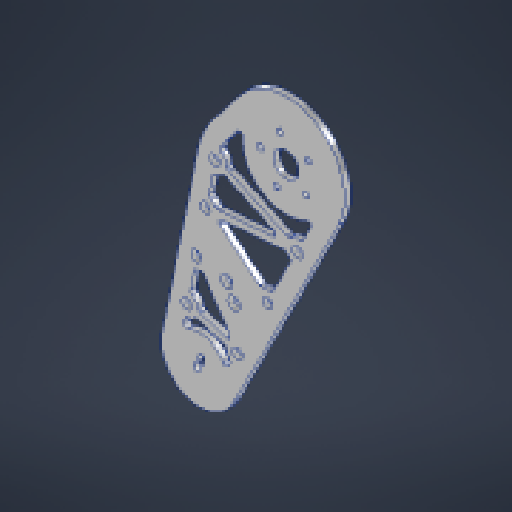
# Autodesk Inventor part: tank_inside_panel
Saved by Autodesk Inventor 2023 (Build 270158000, 158)
## iProperties
Created: 2023-02-28
Part Number: tank_inside_panel
Material: Aluminum 6061
Document SubType Name: Modeling
Designer: ralph
Density: 2.7 g/cm^3
Appearance: Aluminum - Flat
Author: ralph
Autodesk Inventor part; units mm, degrees
(part 1 of 3)
ref_plane "YZ Plane" through (0, 0, 0) normal (1, 0, 0) x (0, 1, 0)
ref_plane "XZ Plane" through (0, 0, 0) normal (0, 1, 0) x (-1, 0, 0)
ref_plane "XY Plane" through (0, 0, 0) normal (0, 0, 1) x (1, 0, 0)
sketch "Sketch1" plane through (0, 0, 0) normal (0, 0, 1) x (1, 0, 0)
  circle A0 centre (-51.8103, -146.0138) radius 3.175 projected
  circle A1 centre (-68.3289, -153.0646) radius 3.175 projected
  line L0 (-87.8938, -227.3235) -> (-92.6277, -239.1082) projected
  arc A2 (-98.5201, -236.7413) -> (-92.6277, -239.1082) centre (-95.5739, -237.9247) ccw projected
  line L1 (-98.5201, -236.7413) -> (-93.7862, -224.9565) projected
  arc A3 (-87.8938, -227.3235) -> (-93.7862, -224.9565) centre (-90.84, -226.14) ccw projected
  circle A4 centre (0, 0) radius 13.4937 projected
  line L2 (-56.4256, -250.7609) -> (56.5867, -28.8131) projected
  arc A5 (56.5867, -28.8131) -> (-50.0844, 39.0359) centre (0, 0) ccw projected
  line L3 (-50.0844, 39.0359) -> (-79.8174, 0.8875) projected
  arc A6 (-79.8174, 0.8875) -> (-94.3869, -30.7665) centre (-19.7161, -45.9556) ccw projected
  line L4 (-94.3869, -30.7665) -> (-133.6537, -223.8049) projected
  arc A7 (-133.6537, -223.8049) -> (-56.4256, -250.7609) centre (-93.207, -232.0324) ccw projected
  circle A8 centre (-6.7845, 27.1038) radius 3.175 projected
  circle A9 centre (-27.8737, 1.9231) radius 3.175 projected
  circle A10 centre (23.6807, 14.828) radius 3.175 projected
  circle A11 centre (-10.4424, -25.9152) radius 3.175 projected
  circle A12 centre (21.42, -17.9396) radius 3.175 projected
  circle A13 centre (12.3657, -76.0454) radius 2.413 projected
  circle A14 centre (-19.9049, -139.4226) radius 2.413 projected
  circle A15 centre (-52.1756, -202.7997) radius 2.413 projected
  line L5 (-60.0739, -215.9422) -> (-61.8764, -219.4822) projected
  arc A16 (-67.5559, -219.4407) -> (-61.8764, -219.4822) centre (-64.7057, -218.0416) ccw projected
  arc A17 (-109.9229, -202.7119) -> (-105.4512, -206.2136) centre (-106.8116, -203.3448) ccw projected
  line L6 (-109.9229, -202.7119) -> (-109.1463, -198.894) projected
  arc A18 (-106.2582, -196.3597) -> (-109.1463, -198.894) centre (-106.035, -199.5269) ccw projected
  arc A19 (-106.2582, -196.3597) -> (-98.2131, -192.7137) centre (-107.1508, -183.6911) ccw projected
  line L7 (4.4674, -89.1879) -> (-13.9226, -125.3045) projected
  arc A20 (-64.7826, -204.3336) -> (-60.7577, -212.1612) centre (-52.1756, -202.7997) ccw projected
  arc A21 (-60.0739, -215.9422) -> (-60.7577, -212.1612) centre (-62.9032, -214.5015) ccw projected
  arc A22 (-92.9225, -119.1363) -> (-91.2539, -122.5975) centre (-89.8112, -119.7692) ccw projected
  line L8 (-92.9225, -119.1363) -> (-88.8942, -99.3329) projected
  arc A23 (-86.006, -96.7986) -> (-88.8942, -99.3329) centre (-85.7829, -99.9658) ccw projected
  arc A24 (-86.006, -96.7986) -> (-81.66, -95.6992) centre (-86.8987, -84.1301) ccw projected
  arc A25 (-82.7964, -69.3558) -> (-81.1278, -72.8169) centre (-79.6851, -69.9886) ccw projected
  line L9 (-82.7964, -69.3558) -> (-78.7681, -49.5524) projected
  arc A26 (-75.88, -47.0181) -> (-78.7681, -49.5524) centre (-75.6568, -50.1853) ccw projected
  arc A27 (-64.0747, -34.1201) -> (-69.5394, -23.9106) centre (-76.7726, -34.3495) ccw projected
  arc A28 (-70.5555, -19.8506) -> (-69.5394, -23.9106) centre (-67.7311, -21.3009) ccw projected
  arc A29 (-64.7921, -10.8233) -> (-70.5555, -19.8506) centre (-19.7161, -45.9556) ccw projected
  line L10 (-64.7921, -10.8233) -> (-52.5862, 4.8373) projected
  arc A30 (-46.9122, 2.7029) -> (-52.5862, 4.8373) centre (-50.0819, 2.8855) ccw projected
  arc A31 (-46.9122, 2.7029) -> (-23.4162, -40.7399) centre (0, 0) ccw projected
  arc A32 (26.6737, -45.5765) -> (22.3352, -41.3425) centre (23.8443, -44.1359) ccw projected
  line L11 (26.6737, -45.5765) -> (18.3481, -61.9274) projected
  arc A33 (14.8881, -63.5984) -> (18.3481, -61.9274) centre (15.5187, -60.4867) ccw projected
  arc A34 (1.4524, -82.5408) -> (3.7836, -85.4069) centre (12.3657, -76.0454) ccw projected
  arc A35 (4.4674, -89.1879) -> (3.7836, -85.4069) centre (1.6381, -87.7473) ccw projected
  arc A36 (-17.3825, -126.9756) -> (-13.9226, -125.3045) centre (-16.7519, -123.8638) ccw projected
  arc A37 (-17.3825, -126.9756) -> (-25.1437, -127.8534) centre (-19.9049, -139.4226) ccw projected
  arc A38 (-63.388, -164.764) -> (-63.3432, -164.745) centre (-68.3289, -153.0646) ccw projected
  line L12 (-63.3432, -164.745) -> (-46.8246, -157.6942) projected
  arc A39 (-46.8246, -157.6942) -> (-39.1239, -145.4255) centre (-51.8103, -146.0138) ccw projected
  arc A40 (-35.726, -142.1115) -> (-39.1239, -145.4255) centre (-35.9523, -145.2784) ccw projected
  line L13 (-35.726, -142.1115) -> (-34.396, -142.2066) projected
  arc A41 (-31.6788, -144.1833) -> (-34.396, -142.2066) centre (-34.6223, -145.3735) ccw projected
  arc A42 (-31.6788, -144.1833) -> (-28.487, -148.784) centre (-19.9049, -139.4226) ccw projected
  arc A43 (-27.8032, -152.5651) -> (-28.487, -148.784) centre (-30.6326, -151.1244) ccw projected
  line L14 (-27.8032, -152.5651) -> (-46.1932, -188.6816) projected
  arc A44 (-49.6531, -190.3527) -> (-46.1932, -188.6816) centre (-49.0225, -187.241) ccw projected
  arc A45 (-49.6531, -190.3527) -> (-50.0187, -190.2842) centre (-52.1756, -202.7997) ccw projected
  arc A46 (-52.1403, -188.8876) -> (-50.0187, -190.2842) centre (-49.4795, -187.1553) ccw projected
  line L15 (-52.1403, -188.8876) -> (-64.8136, -169.4212) projected
  arc A47 (-63.388, -164.764) -> (-64.8136, -169.4212) centre (-62.1528, -167.6889) ccw projected
  arc A48 (-49.8906, -133.4597) -> (-51.925, -133.3143) centre (-51.8103, -146.0138) ccw projected
  line L16 (-51.925, -133.3143) -> (-82.5337, -131.1266) projected
  arc A49 (-85.2508, -129.1499) -> (-82.5337, -131.1266) centre (-82.3074, -127.9597) ccw projected
  arc A50 (-85.2508, -129.1499) -> (-91.2539, -122.5975) centre (-97.0248, -133.9106) ccw projected
  line L17 (-78.3293, -96.1428) -> (-39.1869, -128.4485) projected
  arc A51 (-41.4343, -134.0641) -> (-39.1869, -128.4485) centre (-41.2079, -130.8972) ccw projected
  line L18 (-41.4343, -134.0641) -> (-49.8906, -133.4597) projected
  line L19 (-94.9362, -191.9703) -> (-86.0453, -195.0607) projected
  arc A52 (-64.7826, -204.3336) -> (-66.8919, -201.7181) centre (-67.9343, -204.7171) ccw projected
  arc A53 (-94.9362, -191.9703) -> (-98.2131, -192.7137) centre (-95.9786, -194.9693) ccw projected
  line L20 (-65.4741, -43.8408) -> (-13.0902, -68.3442) projected
  arc A54 (-14.1778, -74.3847) -> (-13.0902, -68.3442) centre (-14.4355, -71.2201) ccw projected
  line L21 (-14.1778, -74.3847) -> (-72.9993, -79.1754) projected
  arc A55 (-75.9854, -77.6347) -> (-72.9993, -79.1754) centre (-73.2571, -76.0109) ccw projected
  arc A56 (-75.9854, -77.6347) -> (-81.1278, -72.8169) centre (-86.8987, -84.1301) ccw projected
  arc A57 (-65.4741, -43.8408) -> (-68.81, -44.2433) centre (-66.8194, -46.7167) ccw projected
  line L22 (-28.4744, -127.4098) -> (-71.2033, -92.144) projected
  arc A58 (-69.4401, -86.5307) -> (-71.2033, -92.144) centre (-69.1823, -89.6953) ccw projected
  line L23 (-69.4401, -86.5307) -> (-1.5337, -81.0001) projected
  arc A59 (1.4524, -82.5408) -> (-1.5337, -81.0001) centre (-1.2759, -84.1646) ccw projected
  arc A60 (-28.4744, -127.4098) -> (-25.1437, -127.8534) centre (-26.4534, -124.9611) ccw projected
  arc A61 (14.8881, -63.5984) -> (4.4031, -66.1517) centre (12.3657, -76.0454) ccw projected
  arc A62 (1.0672, -66.5541) -> (4.4031, -66.1517) centre (2.4124, -63.6782) ccw projected
  line L24 (1.0672, -66.5541) -> (-16.1602, -58.4958) projected
  arc A63 (-64.0747, -34.1201) -> (-62.2455, -36.9386) centre (-60.9002, -34.0627) ccw projected
  arc A64 (-61.0933, -193.7573) -> (-61.1133, -193.7771) centre (-52.1756, -202.7997) ccw projected
  arc A65 (-64.3902, -194.5205) -> (-61.1133, -193.7771) centre (-63.3478, -191.5215) ccw projected
  line L25 (-64.3902, -194.5205) -> (-92.4345, -184.7727) projected
  arc A66 (-94.5438, -182.1572) -> (-92.4345, -184.7727) centre (-91.3921, -181.7737) ccw projected
  arc A67 (-94.5438, -182.1572) -> (-101.38, -172.378) centre (-107.1508, -183.6911) ccw projected
  arc A68 (-103.0485, -168.9169) -> (-101.38, -172.378) centre (-99.9372, -169.5497) ccw projected
  line L26 (-103.0485, -168.9169) -> (-99.0202, -149.1135) projected
  arc A69 (-96.1321, -146.5792) -> (-99.0202, -149.1135) centre (-95.909, -149.7463) ccw projected
  arc A70 (-96.1321, -146.5792) -> (-92.3643, -145.7246) centre (-97.0248, -133.9106) ccw projected
  arc A71 (-88.5384, -146.9458) -> (-92.3643, -145.7246) centre (-91.1992, -148.6781) ccw projected
  line L27 (-88.5384, -146.9458) -> (-60.6619, -189.7645) projected
  arc A72 (-61.0933, -193.7573) -> (-60.6619, -189.7645) centre (-63.3227, -191.4968) ccw projected
  arc A73 (-88.6501, -203.823) -> (-105.4512, -206.2136) centre (-93.207, -232.0324) ccw projected
  line L28 (-22.0522, -44.6761) -> (-24.5423, -50.875) projected
  line L29 (-28.8338, -52.5675) -> (-62.2455, -36.9386) projected
  line L30 (-84.1415, -199.2432) -> (-85.1976, -201.8722) projected
  line L31 (-17.7611, -54.4364) -> (-14.9814, -47.5164) projected
  line L32 (-72.8348, -199.6524) -> (-66.8919, -201.7181) projected
  arc A74 (-67.5559, -219.4407) -> (-76.9832, -208.5096) centre (-93.207, -232.0324) ccw projected
  arc A75 (-75.88, -47.0181) -> (-68.81, -44.2433) centre (-76.7726, -34.3495) ccw projected
  line L33 (-78.1267, -204.7125) -> (-76.8234, -201.468) projected
  arc A76 (-11.2735, -45.6176) -> (22.3352, -41.3425) centre (0, 0) ccw projected
  arc A77 (-84.1415, -199.2432) -> (-86.0453, -195.0607) centre (-87.0877, -198.0597) ccw projected
  arc A78 (-88.6501, -203.823) -> (-85.1976, -201.8722) centre (-88.1438, -200.6887) ccw projected
  arc A79 (-22.0522, -44.6761) -> (-23.4162, -40.7399) centre (-24.9984, -43.4926) ccw projected
  arc A80 (-28.8338, -52.5675) -> (-24.5423, -50.875) centre (-27.4885, -49.6916) ccw projected
  arc A81 (-78.3293, -96.1428) -> (-81.66, -95.6992) centre (-80.3503, -98.5915) ccw projected
  arc A82 (-72.8348, -199.6524) -> (-76.8234, -201.468) centre (-73.8772, -202.6514) ccw projected
  arc A83 (-78.1267, -204.7125) -> (-76.9832, -208.5096) centre (-75.1805, -205.896) ccw projected
  arc A84 (-11.2735, -45.6176) -> (-14.9814, -47.5164) centre (-12.0352, -48.6999) ccw projected
  arc A85 (-17.7611, -54.4364) -> (-16.1602, -58.4958) centre (-14.8149, -55.6198) ccw projected
  point P0 (0, 0)
  point P1 (-30.4878, -157.8365)
  point P2 (-86.8989, -84.1298)
  point P3 (-76.7727, -34.3493)
  point P4 (-67.7312, -21.3007)
  point P5 (0, 0)
  constraints: 1 other
extrude "Extrusion1" add sketch "Sketch1" along normal blind 6.35 contours A7 L4 A6 L3 A5 L2 | A8 | A9 | A10 | A11 | A12 | A13 | A14 | A15 | L5 A16 A74 A83 L33 A82 L32 A52 A20 A21 | L6 A18 A19 A53 L19 A77 L30 A78 A73 A17 | L7 A36 A37 A60 L22 A58 L23 A59 A34 A35 | L8 A23 A24 A81 L17 A51 L18 A48 L16 A49 A50 A22 | L9 A26 A75 A57 L20 A54 L21 A55 A56 A25 | A27 A28 A29 L10 A30 A31 A79 L28 A80 L29 A63 | L11 A33 A61 A62 L24 A85 L31 A84 A76 A32 | A38 L12 A39 A40 L13 A41 A42 A43 L14 A44 A45 A46 L15 A47 | A64 A65 L25 A66 A67 A68 L26 A69 A70 A71 L27 A72
sketch "Sketch2" plane through (0, 0, 6.35) normal (0, 0, 1) x (1, 0, 0)
  line L0 (-92.6277, -239.1082) -> (-87.8938, -227.3235) projected
  arc A0 (-87.8938, -227.3235) -> (-93.7862, -224.9565) centre (-90.84, -226.14) ccw projected
  line L1 (-93.7862, -224.9565) -> (-98.5201, -236.7413) projected
  arc A1 (-98.5201, -236.7413) -> (-92.6277, -239.1082) centre (-95.5739, -237.9247) ccw projected
  circle A2 centre (0, 0) radius 13.4937 projected
  line L2 (-56.4256, -250.7609) -> (56.5867, -28.8131) projected
  arc A3 (-133.6537, -223.8049) -> (-56.4256, -250.7609) centre (-93.207, -232.0324) ccw projected
  line L3 (-94.3869, -30.7665) -> (-133.6537, -223.8049) projected
  arc A4 (-79.8174, 0.8875) -> (-94.3869, -30.7665) centre (-19.7161, -45.9556) ccw projected
  line L4 (-50.0844, 39.0359) -> (-79.8174, 0.8875) projected
  arc A5 (56.5867, -28.8131) -> (-50.0844, 39.0359) centre (0, 0) ccw projected
  circle A6 centre (-10.4424, -25.9152) radius 6.731 projected
  circle A7 centre (-6.7845, 27.1038) radius 6.731 projected
  circle A8 centre (-51.8103, -146.0138) radius 6.731 projected
  circle A9 centre (-68.3289, -153.0646) radius 6.731 projected
  circle A10 centre (23.6807, 14.828) radius 6.731 projected
  circle A11 centre (-27.8737, 1.9231) radius 6.731 projected
  circle A12 centre (21.42, -17.9396) radius 6.731 projected
  circle A13 centre (-19.9051, -139.4228) radius 5.588 projected
  circle A14 centre (-52.1757, -202.7999) radius 5.588 projected
  circle A15 centre (12.3656, -76.0457) radius 5.588 projected
  arc A16 (-64.7827, -204.3338) -> (-60.7578, -212.1614) centre (-52.1757, -202.7999) ccw projected
  line L5 (18.348, -61.9276) -> (26.6737, -45.5765) projected
  arc A17 (-94.5438, -182.1573) -> (-101.38, -172.378) centre (-107.1508, -183.6911) ccw projected
  arc A18 (-106.2582, -196.3597) -> (-109.1463, -198.894) centre (-106.035, -199.5269) ccw projected
  line L6 (-109.1463, -198.894) -> (-109.9229, -202.7119) projected
  arc A19 (-109.9229, -202.7119) -> (-105.4512, -206.2136) centre (-106.8116, -203.3448) ccw projected
  arc A20 (-67.5559, -219.4407) -> (-61.8764, -219.4822) centre (-64.7057, -218.0416) ccw projected
  line L7 (-61.8764, -219.4822) -> (-60.074, -215.9425) projected
  arc A21 (-60.074, -215.9425) -> (-60.7578, -212.1614) centre (-62.9033, -214.5018) ccw projected
  arc A22 (-17.3826, -126.9758) -> (-25.1438, -127.8536) centre (-19.9051, -139.4228) ccw projected
  arc A23 (-17.3826, -126.9758) -> (-13.9227, -125.3047) centre (-16.752, -123.8641) ccw projected
  line L8 (-13.9227, -125.3047) -> (4.4673, -89.1882) projected
  arc A24 (4.4673, -89.1882) -> (3.7835, -85.4072) centre (1.638, -87.7475) ccw projected
  arc A25 (14.888, -63.5987) -> (4.403, -66.1519) centre (12.3656, -76.0457) ccw projected
  arc A26 (14.888, -63.5987) -> (18.348, -61.9276) centre (15.5186, -60.487) ccw projected
  arc A27 (26.6737, -45.5765) -> (22.3352, -41.3425) centre (23.8443, -44.1359) ccw projected
  arc A28 (-11.2735, -45.6176) -> (22.3352, -41.3425) centre (0, 0) ccw projected
  arc A29 (-46.9122, 2.7029) -> (-52.5862, 4.8373) centre (-50.0819, 2.8855) ccw projected
  line L9 (-52.5862, 4.8373) -> (-64.7921, -10.8233) projected
  arc A30 (-64.7921, -10.8233) -> (-70.5555, -19.8506) centre (-19.7161, -45.9556) ccw projected
  arc A31 (-70.5555, -19.8506) -> (-69.5394, -23.9106) centre (-67.7311, -21.3009) ccw projected
  arc A32 (-64.0747, -34.1201) -> (-69.5394, -23.9106) centre (-76.7726, -34.3495) ccw projected
  arc A33 (-75.88, -47.0181) -> (-78.7681, -49.5524) centre (-75.6568, -50.1853) ccw projected
  line L10 (-78.7681, -49.5524) -> (-82.7964, -69.3558) projected
  arc A34 (-82.7964, -69.3558) -> (-81.1278, -72.8169) centre (-79.6851, -69.9886) ccw projected
  arc A35 (-86.006, -96.7986) -> (-81.66, -95.6992) centre (-86.8987, -84.1301) ccw projected
  arc A36 (-86.006, -96.7986) -> (-88.8942, -99.3329) centre (-85.7829, -99.9658) ccw projected
  line L11 (-88.8942, -99.3329) -> (-92.9225, -119.1363) projected
  arc A37 (-92.9225, -119.1363) -> (-91.2539, -122.5975) centre (-89.8112, -119.7692) ccw projected
  line L12 (-60.662, -189.7647) -> (-88.5384, -146.9458) projected
  arc A38 (-88.5384, -146.9458) -> (-92.3643, -145.7246) centre (-91.1992, -148.6781) ccw projected
  arc A39 (-96.1321, -146.5792) -> (-92.3643, -145.7246) centre (-97.0248, -133.9106) ccw projected
  arc A40 (-96.1321, -146.5792) -> (-99.0202, -149.1135) centre (-95.909, -149.7463) ccw projected
  line L13 (-99.0202, -149.1135) -> (-103.0485, -168.9169) projected
  arc A41 (-103.0485, -168.9169) -> (-101.38, -172.378) centre (-99.9372, -169.5497) ccw projected
  arc A42 (-94.5438, -182.1573) -> (-92.4345, -184.7728) centre (-91.3921, -181.7738) ccw projected
  line L14 (-92.4345, -184.7728) -> (-64.3903, -194.5207) projected
  arc A43 (-64.3903, -194.5207) -> (-61.1134, -193.7773) centre (-63.3478, -191.5217) ccw projected
  arc A44 (-61.0934, -193.7576) -> (-61.1134, -193.7773) centre (-52.1757, -202.7999) ccw projected
  arc A45 (-61.0934, -193.7576) -> (-60.662, -189.7647) centre (-63.3228, -191.497) ccw projected
  line L15 (-39.187, -128.4486) -> (-78.3293, -96.1428) projected
  arc A46 (-85.2508, -129.1499) -> (-91.2539, -122.5975) centre (-97.0248, -133.9106) ccw projected
  arc A47 (-85.2508, -129.1499) -> (-82.5337, -131.1266) centre (-82.3073, -127.9597) ccw projected
  line L16 (-82.5337, -131.1266) -> (-51.927, -133.3143) projected
  arc A48 (-49.8886, -133.46) -> (-51.927, -133.3143) centre (-51.8103, -146.0138) ccw projected
  line L17 (-49.8886, -133.46) -> (-41.4344, -134.0643) projected
  arc A49 (-41.4344, -134.0643) -> (-39.187, -128.4486) centre (-41.208, -130.8973) ccw projected
  line L18 (-34.3961, -142.2068) -> (-35.726, -142.1117) projected
  arc A50 (-35.726, -142.1117) -> (-39.1239, -145.4257) centre (-35.9523, -145.2786) ccw projected
  arc A51 (-46.8246, -157.6942) -> (-39.1239, -145.4257) centre (-51.8103, -146.0138) ccw projected
  line L19 (-46.8246, -157.6942) -> (-63.3432, -164.745) projected
  arc A52 (-63.3881, -164.7641) -> (-63.3432, -164.745) centre (-68.3289, -153.0646) ccw projected
  arc A53 (-63.3881, -164.7641) -> (-64.8137, -169.4212) centre (-62.1529, -167.689) ccw projected
  line L20 (-64.8137, -169.4212) -> (-52.1404, -188.8878) projected
  arc A54 (-52.1404, -188.8878) -> (-50.0188, -190.2844) centre (-49.4795, -187.1556) ccw projected
  arc A55 (-49.6533, -190.353) -> (-50.0188, -190.2844) centre (-52.1757, -202.7999) ccw projected
  arc A56 (-49.6533, -190.353) -> (-46.1933, -188.6819) centre (-49.0227, -187.2412) ccw projected
  line L21 (-46.1933, -188.6819) -> (-27.8033, -152.5653) projected
  arc A57 (-27.8033, -152.5653) -> (-28.4872, -148.7843) centre (-30.6327, -151.1247) ccw projected
  arc A58 (-31.679, -144.1835) -> (-28.4872, -148.7843) centre (-19.9051, -139.4228) ccw projected
  arc A59 (-31.679, -144.1835) -> (-34.3961, -142.2068) centre (-34.6225, -145.3737) ccw projected
  arc A60 (-106.2582, -196.3597) -> (-98.2131, -192.7137) centre (-107.1508, -183.6911) ccw projected
  arc A61 (-64.7827, -204.3338) -> (-66.8921, -201.7183) centre (-67.9345, -204.7173) ccw projected
  line L22 (-86.0453, -195.0608) -> (-94.9363, -191.9704) projected
  arc A62 (-94.9363, -191.9704) -> (-98.2131, -192.7137) centre (-95.9787, -194.9694) ccw projected
  line L23 (-16.1602, -58.4959) -> (1.0671, -66.5544) projected
  arc A63 (1.0671, -66.5544) -> (4.403, -66.1519) centre (2.4123, -63.6784) ccw projected
  arc A64 (-64.0747, -34.1201) -> (-62.2455, -36.9386) centre (-60.9002, -34.0627) ccw projected
  arc A65 (-75.88, -47.0181) -> (-68.81, -44.2433) centre (-76.7726, -34.3495) ccw projected
  arc A66 (-75.9854, -77.6347) -> (-81.1278, -72.8169) centre (-86.8987, -84.1301) ccw projected
  arc A67 (-75.9854, -77.6347) -> (-72.9993, -79.1754) centre (-73.257, -76.0109) ccw projected
  line L24 (-72.9993, -79.1754) -> (-14.1779, -74.3848) projected
  arc A68 (-14.1779, -74.3848) -> (-13.0903, -68.3444) centre (-14.4356, -71.2203) ccw projected
  line L25 (-13.0903, -68.3444) -> (-65.4741, -43.8408) projected
  arc A69 (-65.4741, -43.8408) -> (-68.81, -44.2433) centre (-66.8194, -46.7168) ccw projected
  arc A70 (1.4522, -82.541) -> (3.7835, -85.4072) centre (12.3656, -76.0457) ccw projected
  arc A71 (1.4522, -82.541) -> (-1.5338, -81.0003) centre (-1.2761, -84.1648) ccw projected
  line L26 (-1.5338, -81.0003) -> (-69.4401, -86.5308) projected
  arc A72 (-69.4401, -86.5308) -> (-71.2034, -92.144) centre (-69.1824, -89.6953) ccw projected
  line L27 (-71.2034, -92.144) -> (-28.4745, -127.41) projected
  arc A73 (-28.4745, -127.41) -> (-25.1438, -127.8536) centre (-26.4534, -124.9613) ccw projected
  arc A74 (-67.5559, -219.4407) -> (-76.9832, -208.5096) centre (-93.207, -232.0324) ccw projected
  line L28 (-66.8921, -201.7183) -> (-72.8349, -199.6526) projected
  line L29 (-14.9814, -47.5164) -> (-17.7612, -54.4365) projected
  line L30 (-76.8235, -201.4681) -> (-78.1267, -204.7125) projected
  line L31 (-24.5424, -50.8752) -> (-22.0522, -44.6761) projected
  arc A75 (-88.6501, -203.823) -> (-105.4512, -206.2136) centre (-93.207, -232.0324) ccw projected
  line L32 (-85.1976, -201.8722) -> (-84.1416, -199.2433) projected
  arc A76 (-46.9122, 2.7029) -> (-23.4162, -40.7399) centre (0, 0) ccw projected
  line L33 (-62.2455, -36.9386) -> (-28.8338, -52.5676) projected
  arc A77 (-72.8349, -199.6526) -> (-76.8235, -201.4681) centre (-73.8773, -202.6516) ccw projected
  arc A78 (-78.1267, -204.7125) -> (-76.9832, -208.5096) centre (-75.1805, -205.896) ccw projected
  arc A79 (-11.2735, -45.6176) -> (-14.9814, -47.5164) centre (-12.0352, -48.6999) ccw projected
  arc A80 (-17.7612, -54.4365) -> (-16.1602, -58.4959) centre (-14.815, -55.62) ccw projected
  arc A81 (-78.3293, -96.1428) -> (-81.66, -95.6992) centre (-80.3503, -98.5915) ccw projected
  arc A82 (-84.1416, -199.2433) -> (-86.0453, -195.0608) centre (-87.0877, -198.0598) ccw projected
  arc A83 (-88.6501, -203.823) -> (-85.1976, -201.8722) centre (-88.1438, -200.6887) ccw projected
  arc A84 (-22.0522, -44.6761) -> (-23.4162, -40.7399) centre (-24.9984, -43.4926) ccw projected
  arc A85 (-28.8338, -52.5676) -> (-24.5424, -50.8752) centre (-27.4886, -49.6917) ccw projected
  point P0 (0, 0)
  point P1 (-30.4878, -157.8365)
  point P2 (-86.8983, -84.1302)
  point P3 (0.0004, -0.0002)
  constraints: 1 other
extrude "Extrusion2" [suppressed]
sketch "Sketch3" plane through (0, 0, 6.35) normal (0, 0, 1) x (1, 0, 0)
  arc A0 (56.5867, -28.8131) -> (-50.0844, 39.0359) centre (0, 0) ccw projected
  line L0 (-50.0844, 39.0359) -> (-79.8174, 0.8875) projected
  arc A1 (-79.8174, 0.8875) -> (-94.3869, -30.7665) centre (-19.7161, -45.9556) ccw projected
  line L1 (-94.3869, -30.7665) -> (-133.6537, -223.8049) projected
  arc A2 (-133.6537, -223.8049) -> (-56.4256, -250.7609) centre (-93.207, -232.0324) ccw projected
  line L2 (-56.4256, -250.7609) -> (56.5867, -28.8131) projected
  circle A3 centre (-51.8103, -146.0138) radius 3.175 projected
  circle A4 centre (-68.3289, -153.0646) radius 3.175 projected
  circle A5 centre (0, 0) radius 13.4937 projected
  line L3 (-98.5201, -236.7413) -> (-93.7862, -224.9565) projected
  arc A6 (-87.8938, -227.3235) -> (-93.7862, -224.9565) centre (-90.84, -226.14) ccw projected
  line L4 (-87.8938, -227.3235) -> (-92.6277, -239.1082) projected
  arc A7 (-98.5201, -236.7413) -> (-92.6277, -239.1082) centre (-95.5739, -237.9247) ccw projected
  circle A8 centre (-51.8103, -146.0138) radius 3.175 projected
  line L5 (-51.8103, -146.0138) -> (-63.595, -141.2799)
  line L6 (-63.595, -141.2799) -> (-68.3289, -153.0646)
  line L7 (-51.8103, -146.0138) -> (-56.5442, -157.7985)
  line L8 (-56.5442, -157.7985) -> (-68.3289, -153.0646)
  circle A9 centre (-56.5442, -157.7985) radius 3.175
  circle A10 centre (-63.595, -141.2799) radius 3.175
  point P0 (0, 0)
  dimension "d4" = 6.35
  dimension "d5" = 6.35
  constraints: 8 end point, 4 perpendicular, 2 centre point, 2 coincident
  measures "d4" diameter of A9
  measures "d5" diameter of A10
extrude "Extrusion3" cut sketch "Sketch3" against normal blind 6.35 contours A10 L6 L5 | L5 L6 A10 | A9 L8 L7 | L7 L8 A9
sketch "Sketch4" plane through (0, 0, 6.35) normal (0, 0, 1) x (1, 0, 0)
  circle A0 centre (-56.5442, -157.7985) radius 3.175 projected
  circle A1 centre (-63.595, -141.2799) radius 3.175 projected
  arc A2 (56.5867, -28.8131) -> (-50.0844, 39.0359) centre (0, 0) ccw projected
  line L0 (-50.0844, 39.0359) -> (-79.8174, 0.8875) projected
  arc A3 (-79.8174, 0.8875) -> (-94.3869, -30.7665) centre (-19.7161, -45.9556) ccw projected
  line L1 (-94.3869, -30.7665) -> (-133.6537, -223.8049) projected
  arc A4 (-133.6537, -223.8049) -> (-56.4256, -250.7609) centre (-93.207, -232.0324) ccw projected
  line L2 (-56.4256, -250.7609) -> (56.5867, -28.8131) projected
  circle A5 centre (-51.8103, -146.0138) radius 3.175 projected
  circle A6 centre (-68.3289, -153.0646) radius 3.175 projected
  circle A7 centre (0, 0) radius 13.4937 projected
  line L3 (-98.5201, -236.7413) -> (-93.7862, -224.9565) projected
  arc A8 (-87.8938, -227.3235) -> (-93.7862, -224.9565) centre (-90.84, -226.14) ccw projected
  line L4 (-87.8938, -227.3235) -> (-92.6277, -239.1082) projected
  arc A9 (-98.5201, -236.7413) -> (-92.6277, -239.1082) centre (-95.5739, -237.9247) ccw projected
  point P0 (0, 0)
extrude "Extrusion4" add sketch "Sketch4" against normal blind 6.35 contours A5 | A6
chamfer "Chamfer1" distance 3.556 angle 45 2 edges at (-66.77, -141.2799, 6.35) (-59.7192, -157.7985, 6.35)
sketch "Sketch5" plane through (0, 0, 6.35) normal (0, 0, 1) x (1, 0, 0)
  circle A0 centre (-10.4424, -25.9152) radius 6.731 projected
  circle A1 centre (-6.7845, 27.1038) radius 6.731 projected
  circle A2 centre (-51.8103, -146.0138) radius 6.731 projected
  line L0 (-56.4256, -250.7609) -> (56.5867, -28.8131) projected
  arc A3 (-133.6537, -223.8049) -> (-56.4256, -250.7609) centre (-93.207, -232.0324) ccw projected
  line L1 (-94.3869, -30.7665) -> (-133.6537, -223.8049) projected
  arc A4 (-79.8174, 0.8875) -> (-94.3869, -30.7665) centre (-19.7161, -45.9556) ccw projected
  line L2 (-50.0844, 39.0359) -> (-79.8174, 0.8875) projected
  arc A5 (56.5867, -28.8131) -> (-50.0844, 39.0359) centre (0, 0) ccw projected
  circle A6 centre (0, 0) radius 13.4937 projected
  line L3 (-92.6277, -239.1082) -> (-87.8938, -227.3235) projected
  arc A7 (-87.8938, -227.3235) -> (-93.7862, -224.9565) centre (-90.84, -226.14) ccw projected
  line L4 (-93.7862, -224.9565) -> (-98.5201, -236.7413) projected
  arc A8 (-98.5201, -236.7413) -> (-92.6277, -239.1082) centre (-95.5739, -237.9247) ccw projected
  circle A9 centre (-68.3289, -153.0646) radius 6.731 projected
  circle A10 centre (23.6807, 14.828) radius 6.731 projected
  circle A11 centre (-27.8737, 1.9231) radius 6.731 projected
  circle A12 centre (21.42, -17.9396) radius 6.731 projected
  line L5 (-56.4256, -250.7609) -> (56.5867, -28.8131) projected
  arc A13 (56.5867, -28.8131) -> (-50.0844, 39.0359) centre (0, 0) ccw projected
  line L6 (-50.0844, 39.0359) -> (-79.8174, 0.8875) projected
  arc A14 (-79.8174, 0.8875) -> (-94.3869, -30.7665) centre (-19.7161, -45.9556) ccw projected
  line L7 (-94.3869, -30.7665) -> (-133.6537, -223.8049) projected
  arc A15 (-133.6537, -223.8049) -> (-56.4256, -250.7609) centre (-93.207, -232.0324) ccw projected
  circle A16 centre (0, 0) radius 13.4937 projected
  line L8 (-87.8938, -227.3235) -> (-92.6277, -239.1082) projected
  arc A17 (-98.5201, -236.7413) -> (-92.6277, -239.1082) centre (-95.5739, -237.9247) ccw projected
  line L9 (-98.5201, -236.7413) -> (-93.7862, -224.9565) projected
  arc A18 (-87.8938, -227.3235) -> (-93.7862, -224.9565) centre (-90.84, -226.14) ccw projected
  circle A19 centre (-68.3289, -153.0646) radius 3.175 projected
  circle A20 centre (-51.8103, -146.0138) radius 3.175 projected
  arc A21 (23.8681, -19.9613) -> (18.9971, -15.8876) centre (21.4452, -17.9094) ccw projected
  arc A22 (18.9971, -15.8876) -> (23.8681, -19.9613) centre (21.42, -17.9396) ccw projected
  arc A23 (-11.6087, -28.8683) -> (-9.2396, -22.9769) centre (-10.4059, -25.9299) ccw projected
  arc A24 (-9.2396, -22.9769) -> (-11.6087, -28.8683) centre (-10.4424, -25.9152) ccw projected
  arc A25 (26.36, 16.5315) -> (20.9805, 13.1578) centre (23.6598, 14.8613) ccw projected
  arc A26 (20.9805, 13.1578) -> (26.36, 16.5315) centre (23.6807, 14.828) ccw projected
  arc A27 (-31.0426, 2.1197) -> (-24.7075, 1.6871) centre (-27.8764, 1.8838) ccw projected
  arc A28 (-24.7075, 1.6871) -> (-31.0426, 2.1197) centre (-27.8737, 1.9231) ccw projected
  arc A29 (-7.5767, 30.1783) -> (-6.0305, 24.0196) centre (-6.8227, 27.0942) ccw projected
  arc A30 (-6.0305, 24.0196) -> (-7.5767, 30.1783) centre (-6.7845, 27.1038) ccw projected
  circle A31 centre (-19.9049, -139.4226) radius 5.588 projected
  circle A32 centre (-52.1756, -202.7997) radius 5.588 projected
  circle A33 centre (12.3657, -76.0454) radius 5.588 projected
  circle A34 centre (-52.1757, -202.7999) radius 2.413 projected
  circle A35 centre (-19.9051, -139.4228) radius 2.413 projected
  circle A36 centre (12.3656, -76.0457) radius 2.413 projected
  arc A37 (-64.7826, -204.3336) -> (-60.7577, -212.1612) centre (-52.1756, -202.7997) ccw projected
  line L10 (18.3481, -61.9274) -> (26.6737, -45.5765) projected
  arc A38 (-94.5438, -182.1572) -> (-101.38, -172.378) centre (-107.1508, -183.6911) ccw projected
  arc A39 (-106.2582, -196.3597) -> (-109.1463, -198.894) centre (-106.035, -199.5269) ccw projected
  line L11 (-109.1463, -198.894) -> (-109.9229, -202.7119) projected
  arc A40 (-109.9229, -202.7119) -> (-105.4512, -206.2136) centre (-106.8116, -203.3448) ccw projected
  arc A41 (-67.5559, -219.4407) -> (-61.8764, -219.4822) centre (-64.7057, -218.0416) ccw projected
  line L12 (-61.8764, -219.4822) -> (-60.0739, -215.9422) projected
  arc A42 (-60.0739, -215.9422) -> (-60.7577, -212.1612) centre (-62.9032, -214.5015) ccw projected
  arc A43 (-17.3825, -126.9756) -> (-25.1437, -127.8534) centre (-19.9049, -139.4226) ccw projected
  arc A44 (-17.3825, -126.9756) -> (-13.9226, -125.3045) centre (-16.7519, -123.8638) ccw projected
  line L13 (-13.9226, -125.3045) -> (4.4674, -89.1879) projected
  arc A45 (4.4674, -89.1879) -> (3.7836, -85.4069) centre (1.6381, -87.7473) ccw projected
  arc A46 (14.8881, -63.5984) -> (4.4031, -66.1517) centre (12.3657, -76.0454) ccw projected
  arc A47 (14.8881, -63.5984) -> (18.3481, -61.9274) centre (15.5187, -60.4867) ccw projected
  arc A48 (26.6737, -45.5765) -> (22.3352, -41.3425) centre (23.8443, -44.1359) ccw projected
  arc A49 (-11.2735, -45.6176) -> (22.3352, -41.3425) centre (0, 0) ccw projected
  arc A50 (-46.9122, 2.7029) -> (-52.5862, 4.8373) centre (-50.0819, 2.8855) ccw projected
  line L14 (-52.5862, 4.8373) -> (-64.7921, -10.8233) projected
  arc A51 (-64.7921, -10.8233) -> (-70.5555, -19.8506) centre (-19.7161, -45.9556) ccw projected
  arc A52 (-70.5555, -19.8506) -> (-69.5394, -23.9106) centre (-67.7311, -21.3009) ccw projected
  arc A53 (-64.0747, -34.1201) -> (-69.5394, -23.9106) centre (-76.7726, -34.3495) ccw projected
  arc A54 (-75.88, -47.0181) -> (-78.7681, -49.5524) centre (-75.6568, -50.1853) ccw projected
  line L15 (-78.7681, -49.5524) -> (-82.7964, -69.3558) projected
  arc A55 (-82.7964, -69.3558) -> (-81.1278, -72.8169) centre (-79.6851, -69.9886) ccw projected
  arc A56 (-86.006, -96.7986) -> (-81.66, -95.6992) centre (-86.8987, -84.1301) ccw projected
  arc A57 (-86.006, -96.7986) -> (-88.8942, -99.3329) centre (-85.7829, -99.9658) ccw projected
  line L16 (-88.8942, -99.3329) -> (-92.9225, -119.1363) projected
  arc A58 (-92.9225, -119.1363) -> (-91.2539, -122.5975) centre (-89.8112, -119.7692) ccw projected
  line L17 (-60.6619, -189.7645) -> (-88.5384, -146.9458) projected
  arc A59 (-88.5384, -146.9458) -> (-92.3643, -145.7246) centre (-91.1992, -148.6781) ccw projected
  arc A60 (-96.1321, -146.5792) -> (-92.3643, -145.7246) centre (-97.0248, -133.9106) ccw projected
  arc A61 (-96.1321, -146.5792) -> (-99.0202, -149.1135) centre (-95.909, -149.7463) ccw projected
  line L18 (-99.0202, -149.1135) -> (-103.0485, -168.9169) projected
  arc A62 (-103.0485, -168.9169) -> (-101.38, -172.378) centre (-99.9372, -169.5497) ccw projected
  arc A63 (-94.5438, -182.1572) -> (-92.4345, -184.7727) centre (-91.3921, -181.7737) ccw projected
  line L19 (-92.4345, -184.7727) -> (-64.3902, -194.5205) projected
  arc A64 (-64.3902, -194.5205) -> (-61.1133, -193.7771) centre (-63.3478, -191.5215) ccw projected
  arc A65 (-61.0933, -193.7573) -> (-61.1133, -193.7771) centre (-52.1756, -202.7997) ccw projected
  arc A66 (-61.0933, -193.7573) -> (-60.6619, -189.7645) centre (-63.3227, -191.4968) ccw projected
  line L20 (-39.1869, -128.4485) -> (-78.3293, -96.1428) projected
  arc A67 (-85.2508, -129.1499) -> (-91.2539, -122.5975) centre (-97.0248, -133.9106) ccw projected
  arc A68 (-85.2508, -129.1499) -> (-82.5337, -131.1266) centre (-82.3074, -127.9597) ccw projected
  line L21 (-82.5337, -131.1266) -> (-51.925, -133.3143) projected
  arc A69 (-49.8906, -133.4597) -> (-51.925, -133.3143) centre (-51.8103, -146.0138) ccw projected
  line L22 (-49.8906, -133.4597) -> (-41.4343, -134.0641) projected
  arc A70 (-41.4343, -134.0641) -> (-39.1869, -128.4485) centre (-41.2079, -130.8972) ccw projected
  line L23 (-34.396, -142.2066) -> (-35.726, -142.1115) projected
  arc A71 (-35.726, -142.1115) -> (-39.1239, -145.4255) centre (-35.9523, -145.2784) ccw projected
  arc A72 (-46.8246, -157.6942) -> (-39.1239, -145.4255) centre (-51.8103, -146.0138) ccw projected
  line L24 (-46.8246, -157.6942) -> (-63.3432, -164.745) projected
  arc A73 (-63.388, -164.764) -> (-63.3432, -164.745) centre (-68.3289, -153.0646) ccw projected
  arc A74 (-63.388, -164.764) -> (-64.8136, -169.4212) centre (-62.1528, -167.6889) ccw projected
  line L25 (-64.8136, -169.4212) -> (-52.1403, -188.8876) projected
  arc A75 (-52.1403, -188.8876) -> (-50.0187, -190.2842) centre (-49.4795, -187.1553) ccw projected
  arc A76 (-49.6531, -190.3527) -> (-50.0187, -190.2842) centre (-52.1756, -202.7997) ccw projected
  arc A77 (-49.6531, -190.3527) -> (-46.1932, -188.6816) centre (-49.0225, -187.241) ccw projected
  line L26 (-46.1932, -188.6816) -> (-27.8032, -152.5651) projected
  arc A78 (-27.8032, -152.5651) -> (-28.487, -148.784) centre (-30.6326, -151.1244) ccw projected
  arc A79 (-31.6788, -144.1833) -> (-28.487, -148.784) centre (-19.9049, -139.4226) ccw projected
  arc A80 (-31.6788, -144.1833) -> (-34.396, -142.2066) centre (-34.6223, -145.3735) ccw projected
  arc A81 (-106.2582, -196.3597) -> (-98.2131, -192.7137) centre (-107.1508, -183.6911) ccw projected
  arc A82 (-64.7826, -204.3336) -> (-66.8919, -201.7181) centre (-67.9343, -204.7171) ccw projected
  line L27 (-66.8919, -201.7181) -> (-72.8348, -199.6524) projected
  arc A83 (-94.9362, -191.9703) -> (-98.2131, -192.7137) centre (-95.9786, -194.9693) ccw projected
  line L28 (-62.2455, -36.9386) -> (-28.8338, -52.5675) projected
  arc A84 (1.0672, -66.5541) -> (4.4031, -66.1517) centre (2.4124, -63.6782) ccw projected
  arc A85 (-64.0747, -34.1201) -> (-62.2455, -36.9386) centre (-60.9002, -34.0627) ccw projected
  arc A86 (-75.88, -47.0181) -> (-68.81, -44.2433) centre (-76.7726, -34.3495) ccw projected
  arc A87 (-75.9854, -77.6347) -> (-81.1278, -72.8169) centre (-86.8987, -84.1301) ccw projected
  arc A88 (-75.9854, -77.6347) -> (-72.9993, -79.1754) centre (-73.2571, -76.0109) ccw projected
  line L29 (-72.9993, -79.1754) -> (-14.1778, -74.3847) projected
  arc A89 (-14.1778, -74.3847) -> (-13.0902, -68.3442) centre (-14.4355, -71.2201) ccw projected
  line L30 (-13.0902, -68.3442) -> (-65.4741, -43.8408) projected
  arc A90 (-65.4741, -43.8408) -> (-68.81, -44.2433) centre (-66.8194, -46.7167) ccw projected
  arc A91 (1.4524, -82.5408) -> (3.7836, -85.4069) centre (12.3657, -76.0454) ccw projected
  arc A92 (1.4524, -82.5408) -> (-1.5337, -81.0001) centre (-1.2759, -84.1646) ccw projected
  line L31 (-1.5337, -81.0001) -> (-69.4401, -86.5307) projected
  arc A93 (-69.4401, -86.5307) -> (-71.2033, -92.144) centre (-69.1823, -89.6953) ccw projected
  line L32 (-71.2033, -92.144) -> (-28.4744, -127.4098) projected
  arc A94 (-28.4744, -127.4098) -> (-25.1437, -127.8534) centre (-26.4534, -124.9611) ccw projected
  line L33 (-60.0739, -215.9422) -> (-61.8764, -219.4822) projected
  arc A95 (-67.5559, -219.4407) -> (-61.8764, -219.4822) centre (-64.7057, -218.0416) ccw projected
  arc A96 (-109.9229, -202.7119) -> (-105.4512, -206.2136) centre (-106.8116, -203.3448) ccw projected
  line L34 (-109.9229, -202.7119) -> (-109.1463, -198.894) projected
  arc A97 (-106.2582, -196.3597) -> (-109.1463, -198.894) centre (-106.035, -199.5269) ccw projected
  arc A98 (-106.2582, -196.3597) -> (-98.2131, -192.7137) centre (-107.1508, -183.6911) ccw projected
  line L35 (4.4674, -89.1879) -> (-13.9226, -125.3045) projected
  arc A99 (-64.7827, -204.3338) -> (-60.7578, -212.1614) centre (-52.1757, -202.7999) ccw projected
  arc A100 (-60.0739, -215.9422) -> (-60.7577, -212.1612) centre (-62.9033, -214.5018) ccw projected
  arc A101 (-92.9225, -119.1363) -> (-91.2539, -122.5975) centre (-89.8112, -119.7692) ccw projected
  line L36 (-92.9225, -119.1363) -> (-88.8942, -99.3329) projected
  arc A102 (-86.006, -96.7986) -> (-88.8942, -99.3329) centre (-85.7829, -99.9658) ccw projected
  arc A103 (-86.006, -96.7986) -> (-81.66, -95.6992) centre (-86.8987, -84.1301) ccw projected
  arc A104 (-82.7964, -69.3558) -> (-81.1278, -72.8169) centre (-79.6851, -69.9886) ccw projected
  line L37 (-82.7964, -69.3558) -> (-78.7681, -49.5524) projected
  arc A105 (-75.88, -47.0181) -> (-78.7681, -49.5524) centre (-75.6568, -50.1853) ccw projected
  arc A106 (-64.0747, -34.1201) -> (-69.5394, -23.9106) centre (-76.7726, -34.3495) ccw projected
  arc A107 (-70.5555, -19.8506) -> (-69.5394, -23.9106) centre (-67.7311, -21.3009) ccw projected
  arc A108 (-64.7921, -10.8233) -> (-70.5555, -19.8506) centre (-19.7161, -45.9556) ccw projected
  line L38 (-64.7921, -10.8233) -> (-52.5862, 4.8373) projected
  arc A109 (-46.9122, 2.7029) -> (-52.5862, 4.8373) centre (-50.0819, 2.8855) ccw projected
  arc A110 (-46.9122, 2.7029) -> (-23.4162, -40.7399) centre (0, 0) ccw projected
  arc A111 (26.6737, -45.5765) -> (22.3352, -41.3425) centre (23.8443, -44.1359) ccw projected
  line L39 (26.6737, -45.5765) -> (18.3481, -61.9274) projected
  arc A112 (14.888, -63.5987) -> (18.3481, -61.9274) centre (15.5186, -60.487) ccw projected
  arc A113 (1.4522, -82.541) -> (3.7835, -85.4072) centre (12.3656, -76.0457) ccw projected
  arc A114 (4.4674, -89.1879) -> (3.7836, -85.4069) centre (1.638, -87.7475) ccw projected
  arc A115 (-17.3826, -126.9758) -> (-13.9226, -125.3045) centre (-16.752, -123.8641) ccw projected
  arc A116 (-17.3825, -126.9756) -> (-25.1438, -127.8536) centre (-19.9051, -139.4228) ccw projected
  arc A117 (-63.3881, -164.7641) -> (-63.3432, -164.745) centre (-68.3289, -153.0646) ccw projected
  line L40 (-63.3432, -164.745) -> (-46.8246, -157.6942) projected
  arc A118 (-46.8246, -157.6942) -> (-39.1239, -145.4257) centre (-51.8103, -146.0138) ccw projected
  arc A119 (-35.726, -142.1117) -> (-39.1239, -145.4255) centre (-35.9523, -145.2786) ccw projected
  line L41 (-35.726, -142.1117) -> (-34.396, -142.2068) projected
  arc A120 (-31.679, -144.1835) -> (-34.396, -142.2066) centre (-34.6225, -145.3737) ccw projected
  arc A121 (-31.6788, -144.1833) -> (-28.4872, -148.7843) centre (-19.9051, -139.4228) ccw projected
  arc A122 (-27.8033, -152.5653) -> (-28.487, -148.784) centre (-30.6327, -151.1247) ccw projected
  line L42 (-27.8032, -152.5651) -> (-46.1932, -188.6816) projected
  arc A123 (-49.6533, -190.353) -> (-46.1932, -188.6816) centre (-49.0227, -187.2412) ccw projected
  arc A124 (-49.6531, -190.3527) -> (-50.0188, -190.2844) centre (-52.1757, -202.7999) ccw projected
  arc A125 (-52.1404, -188.8878) -> (-50.0187, -190.2842) centre (-49.4795, -187.1556) ccw projected
  line L43 (-52.1404, -188.8877) -> (-64.8137, -169.4213) projected
  arc A126 (-63.3881, -164.7641) -> (-64.8136, -169.4212) centre (-62.1529, -167.689) ccw projected
  arc A127 (-49.8886, -133.46) -> (-51.927, -133.3143) centre (-51.8103, -146.0138) ccw projected
  line L44 (-51.925, -133.3144) -> (-82.5337, -131.1266) projected
  arc A128 (-85.2508, -129.1499) -> (-82.5337, -131.1266) centre (-82.3073, -127.9597) ccw projected
  arc A129 (-85.2508, -129.1499) -> (-91.2539, -122.5975) centre (-97.0248, -133.9106) ccw projected
  line L45 (-78.3293, -96.1428) -> (-39.1871, -128.4486) projected
  arc A130 (-41.4344, -134.0643) -> (-39.1869, -128.4485) centre (-41.208, -130.8973) ccw projected
  line L46 (-41.4343, -134.0643) -> (-49.8906, -133.4598) projected
  line L47 (-94.9363, -191.9704) -> (-86.0453, -195.0608) projected
  arc A131 (-64.7826, -204.3336) -> (-66.8921, -201.7183) centre (-67.9345, -204.7173) ccw projected
  arc A132 (-94.9362, -191.9703) -> (-98.2131, -192.7137) centre (-95.9787, -194.9694) ccw projected
  line L48 (-65.4741, -43.8408) -> (-13.0903, -68.3444) projected
  arc A133 (-14.1779, -74.3848) -> (-13.0902, -68.3442) centre (-14.4356, -71.2203) ccw projected
  line L49 (-14.1777, -74.3848) -> (-72.9993, -79.1754) projected
  arc A134 (-75.9854, -77.6347) -> (-72.9993, -79.1754) centre (-73.257, -76.0109) ccw projected
  arc A135 (-75.9854, -77.6347) -> (-81.1278, -72.8169) centre (-86.8987, -84.1301) ccw projected
  arc A136 (-65.4741, -43.8408) -> (-68.81, -44.2433) centre (-66.8194, -46.7168) ccw projected
  line L50 (-28.4745, -127.41) -> (-71.2034, -92.144) projected
  arc A137 (-69.4401, -86.5308) -> (-71.2033, -92.144) centre (-69.1824, -89.6953) ccw projected
  line L51 (-69.4401, -86.5308) -> (-1.5337, -81.0003) projected
  arc A138 (1.4524, -82.5408) -> (-1.5337, -81.0001) centre (-1.2761, -84.1648) ccw projected
  arc A139 (-28.4744, -127.4098) -> (-25.1437, -127.8534) centre (-26.4534, -124.9613) ccw projected
  arc A140 (14.8881, -63.5984) -> (4.403, -66.1519) centre (12.3656, -76.0457) ccw projected
  arc A141 (1.0671, -66.5544) -> (4.4031, -66.1517) centre (2.4123, -63.6784) ccw projected
  line L52 (1.0671, -66.5544) -> (-16.1602, -58.4959) projected
  arc A142 (-64.0747, -34.1201) -> (-62.2455, -36.9386) centre (-60.9002, -34.0627) ccw projected
  arc A143 (-61.0934, -193.7576) -> (-61.1134, -193.7773) centre (-52.1757, -202.7999) ccw projected
  arc A144 (-64.3903, -194.5207) -> (-61.1133, -193.7771) centre (-63.3478, -191.5217) ccw projected
  line L53 (-64.3902, -194.5207) -> (-92.4345, -184.7728) projected
  arc A145 (-94.5438, -182.1573) -> (-92.4345, -184.7727) centre (-91.3921, -181.7738) ccw projected
  arc A146 (-94.5438, -182.1573) -> (-101.38, -172.378) centre (-107.1508, -183.6911) ccw projected
  arc A147 (-103.0485, -168.9169) -> (-101.38, -172.378) centre (-99.9372, -169.5497) ccw projected
  line L54 (-103.0485, -168.9169) -> (-99.0202, -149.1135) projected
  arc A148 (-96.1321, -146.5792) -> (-99.0202, -149.1135) centre (-95.909, -149.7463) ccw projected
  arc A149 (-96.1321, -146.5792) -> (-92.3643, -145.7246) centre (-97.0248, -133.9106) ccw projected
  arc A150 (-88.5384, -146.9458) -> (-92.3643, -145.7246) centre (-91.1992, -148.6781) ccw projected
  line L55 (-88.5384, -146.9458) -> (-60.6621, -189.7646) projected
  arc A151 (-61.0933, -193.7573) -> (-60.6619, -189.7645) centre (-63.3228, -191.497) ccw projected
  arc A152 (-67.5559, -219.4407) -> (-76.9832, -208.5096) centre (-93.207, -232.0324) ccw projected
  line L56 (-76.8234, -201.468) -> (-78.1267, -204.7125) projected
  line L57 (-16.1602, -58.4958) -> (1.0672, -66.5541) projected
  line L58 (-14.9814, -47.5164) -> (-17.7611, -54.4364) projected
  line L59 (-85.1976, -201.8722) -> (-84.1415, -199.2432) projected
  line L60 (-86.0453, -195.0607) -> (-94.9362, -191.9703) projected
  arc A153 (-88.6501, -203.823) -> (-105.4512, -206.2136) centre (-93.207, -232.0324) ccw projected
  line L61 (-24.5423, -50.875) -> (-22.0522, -44.6761) projected
  arc A154 (-46.9122, 2.7029) -> (-23.4162, -40.7399) centre (0, 0) ccw projected
  arc A155 (-72.8348, -199.6524) -> (-76.8234, -201.468) centre (-73.8772, -202.6514) ccw projected
  arc A156 (-78.1267, -204.7125) -> (-76.9832, -208.5096) centre (-75.1805, -205.896) ccw projected
  arc A157 (-11.2735, -45.6176) -> (-14.9814, -47.5164) centre (-12.0352, -48.6999) ccw projected
  arc A158 (-17.7611, -54.4364) -> (-16.1602, -58.4958) centre (-14.8149, -55.6198) ccw projected
  arc A159 (-78.3293, -96.1428) -> (-81.66, -95.6992) centre (-80.3503, -98.5915) ccw projected
  arc A160 (-84.1415, -199.2432) -> (-86.0453, -195.0607) centre (-87.0877, -198.0597) ccw projected
  arc A161 (-88.6501, -203.823) -> (-85.1976, -201.8722) centre (-88.1438, -200.6887) ccw projected
  arc A162 (-22.0522, -44.6761) -> (-23.4162, -40.7399) centre (-24.9984, -43.4926) ccw projected
  arc A163 (-28.8338, -52.5675) -> (-24.5423, -50.875) centre (-27.4885, -49.6916) ccw projected
  arc A164 (-88.6501, -203.823) -> (-105.4512, -206.2136) centre (-93.207, -232.0324) ccw projected
  line L62 (-84.1416, -199.2433) -> (-85.1976, -201.8722) projected
  line L63 (-28.8338, -52.5676) -> (-62.2455, -36.9386) projected
  line L64 (-22.0522, -44.6761) -> (-24.5424, -50.8752) projected
  line L65 (-78.1267, -204.7125) -> (-76.8235, -201.4681) projected
  line L66 (-72.8349, -199.6526) -> (-66.8921, -201.7183) projected
  arc A165 (-67.5559, -219.4407) -> (-76.9832, -208.5096) centre (-93.207, -232.0324) ccw projected
  arc A166 (-75.88, -47.0181) -> (-68.81, -44.2433) centre (-76.7726, -34.3495) ccw projected
  line L67 (-17.7612, -54.4365) -> (-14.9814, -47.5164) projected
  arc A167 (-11.2735, -45.6176) -> (22.3352, -41.3425) centre (0, 0) ccw projected
  arc A168 (-84.1416, -199.2433) -> (-86.0453, -195.0607) centre (-87.0877, -198.0598) ccw projected
  arc A169 (-88.6501, -203.823) -> (-85.1976, -201.8722) centre (-88.1438, -200.6887) ccw projected
  arc A170 (-22.0522, -44.6761) -> (-23.4162, -40.7399) centre (-24.9984, -43.4926) ccw projected
  arc A171 (-28.8338, -52.5675) -> (-24.5424, -50.8752) centre (-27.4886, -49.6917) ccw projected
  arc A172 (-78.3293, -96.1428) -> (-81.66, -95.6992) centre (-80.3503, -98.5915) ccw projected
  arc A173 (-72.8348, -199.6524) -> (-76.8234, -201.468) centre (-73.8773, -202.6516) ccw projected
  arc A174 (-78.1267, -204.7125) -> (-76.9832, -208.5096) centre (-75.1805, -205.896) ccw projected
  arc A175 (-11.2735, -45.6176) -> (-14.9814, -47.5164) centre (-12.0352, -48.6999) ccw projected
  arc A176 (-17.7611, -54.4364) -> (-16.1602, -58.4958) centre (-14.815, -55.62) ccw projected
  point P0 (0, 0)
  point P1 (-30.4878, -157.8365)
  point P2 (-86.8989, -84.1298)
  point P3 (-18.5783, -126.792)
  point P4 (-86.8983, -84.1302)
  point P5 (-76.7727, -34.3493)
  point P6 (-67.7312, -21.3007)
  point P7 (0, 0)
  point P8 (-18.8807, -57.2232)
  point P9 (-82.9011, -196.1535)
  point P10 (-20.9933, -42.0397)
  point P11 (0.0004, -0.0002)
  point P12 (-78.3293, -96.1428)
  point P13 (-16.1602, -58.4959)
  constraints: 35 other
extrude "Extrusion5" cut sketch "Sketch5" against normal blind 6.35 contours A22 A21 | A24 A23 | A26 A25 | A28 A27 | A30 A29
sketch "Sketch6" plane through (0, 0, 0) normal (0, 0, -1) x (-1, 0, 0)
  arc A0 (101.216, -186.356) -> (103.586, -188.8104) centre (104.3273, -185.7232) ccw projected
  arc A1 (110.0591, -190.8998) -> (103.586, -188.8104) centre (93.2085, -232.032) ccw projected
  arc A2 (110.0591, -190.8998) -> (114.374, -187.3289) centre (111.2627, -187.9618) ccw projected
  line L0 (114.374, -187.3289) -> (82.9982, -33.0831) projected
  arc A3 (82.9982, -33.0831) -> (70.7531, -6.3888) centre (19.7176, -45.9553) ccw projected
  arc A4 (70.7531, -6.3888) -> (65.1326, -8.9671) centre (68.2439, -8.3342) ccw projected
  line L1 (65.1326, -8.9671) -> (101.216, -186.356) projected
  circle A5 centre (97.0281, -133.9113) radius 2.413 projected
  circle A6 centre (86.902, -84.1308) radius 2.413 projected
  circle A7 centre (107.1541, -183.6919) radius 2.413 projected
  circle A8 centre (76.7759, -34.3502) radius 2.413 projected
  point P0 (0, 0)
extrude "Extrusion6" cut sketch "Sketch6" against normal blind 6.35 contours A5 | A6 | A7 | A8
chamfer "Chamfer3" distance 3.175 angle 45 4 edges at (-74.3629, -34.3502, 6.35) (-84.489, -84.1308, 6.35) (-94.6151, -133.9113, 6.35) (-104.7411, -183.6919, 6.35)
sketch "Sketch7" plane through (0, 0, 6.35) normal (0, 0, 1) x (1, 0, 0)
  circle A0 centre (12.3657, -76.0454) radius 2.413 projected
  circle A1 centre (-52.1756, -202.7997) radius 2.413 projected
  circle A2 centre (-19.9049, -139.4226) radius 2.413 projected
  arc A3 (21.5367, -72.0288) -> (17.894, -67.5191) centre (18.7074, -70.5881) ccw projected
  line L0 (-48.8219, -210.2079) -> (21.5367, -72.0288) projected
  arc A4 (-54.4216, -210.3183) -> (-48.8219, -210.2079) centre (-51.6513, -208.7673) ccw projected
  arc A5 (-54.4216, -210.3183) -> (-58.1887, -204.6549) centre (-93.207, -232.0324) ccw projected
  arc A6 (-58.5167, -201.2588) -> (-58.1887, -204.6549) centre (-55.6874, -202.6994) ccw projected
  line L1 (7.9162, -70.7894) -> (-58.5167, -201.2588) projected
  arc A7 (10.2783, -69.0896) -> (7.9162, -70.7894) centre (10.7455, -72.2301) ccw projected
  arc A8 (10.2783, -69.0896) -> (17.894, -67.5191) centre (0, 0) ccw projected
  point P0 (0, 0)
extrude "Extrusion7" cut sketch "Sketch7" against normal blind 6.35 contours A0 | A1 | A2
chamfer "Chamfer4" distance 3.175 angle 45 3 edges at (9.9527, -76.0454, 6.35) (-22.3179, -139.4226, 6.35) (-54.5886, -202.7997, 6.35)